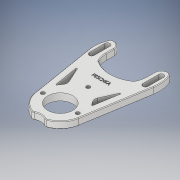
# Autodesk Inventor part: Motor Holder v3
Saved by Autodesk Inventor 2019.3 (Build 233278000, 278)
## iProperties
Created: 2019-03-01
Part Number: Motor Holder v3
Material: ABS Plastic
Document SubType Name: Modeling
Designer: Petar
Density: 1.06 g/cm^3
Appearance: Smooth - White
Mass: 26.5004 g
Surface Area: 70.5339 cm^2
Volume: 9.81495 cm^3
Author: Petar
Autodesk Inventor part; units mm, degrees
ref_plane "YZ Plane" through (0, 0, 0) normal (1, 0, 0) x (0, 1, 0)
ref_plane "XZ Plane" through (0, 0, 0) normal (0, 1, 0) x (-1, 0, 0)
ref_plane "XY Plane" through (0, 0, 0) normal (0, 0, 1) x (1, 0, 0)
sketch "Sketch1" plane through (0, 0, 0) normal (0, 1, 0) x (-1, 0, 0)
  line L0 (0, 0) -> (0, 52.2) construction
  circle A0 centre (0, 52.2) radius 10
  line L1 (16, -6.25) -> (16, 0)
  line L2 (21.2132, 18.9419) -> (21.2132, -15.0581) construction
  line L3 (-21.2132, 18) -> (-21.2132, -16) construction
  circle A1 centre (21.2132, 3.5) radius 1.75 construction
  circle A2 centre (21.2132, -3.5) radius 1.75 construction
  circle A3 centre (-21.2132, 3.5) radius 1.75 construction
  circle A4 centre (-21.2132, -3.5) radius 1.75 construction
  line L4 (-16, -6.25) -> (-16, 0)
  line L5 (21.2132, 6.25) -> (21.2132, -6.25) construction
  line L6 (19.2132, 6.25) -> (19.2132, -6.25)
  line L7 (23.2132, -6.25) -> (23.2132, 6.25)
  arc A5 (23.2132, 6.25) -> (19.2132, 6.25) centre (21.2132, 6.25) ccw
  arc A6 (19.2132, -6.25) -> (23.2132, -6.25) centre (21.2132, -6.25) ccw
  line L8 (-19.2132, 6.25) -> (-19.2132, -6.25)
  line L9 (-23.2132, -6.25) -> (-23.2132, 6.25)
  arc A7 (-19.2132, 6.25) -> (-23.2132, 6.25) centre (-21.2132, 6.25) ccw
  arc A8 (-23.2132, -6.25) -> (-19.2132, -6.25) centre (-21.2132, -6.25) ccw
  arc A9 (14.3275, 42.1515) -> (17.2664, 55.0496) centre (0, 52.2) ccw construction
  arc A10 (16, -6.25) -> (23.6156, -10.8766) centre (21.2132, -6.25) ccw
  arc A11 (-23.6156, -10.8766) -> (-16, -6.25) centre (-21.2132, -6.25) ccw
  line L10 (17.2664, 55.0496) -> (25.653, 4.2337)
  line L11 (-17.2664, 55.0496) -> (-25.653, 4.2337)
  circle A12 centre (0, 52.2) radius 13.75 construction
  circle A13 centre (9.7227, 61.9227) radius 1.5 construction
  circle A14 centre (9.7227, 42.4773) radius 1.5 construction
  line L12 (0, 52.2) -> (9.7227, 61.9227) construction
  line L13 (9.7227, 42.4773) -> (0, 52.2) construction
  circle A15 centre (-9.7227, 61.9227) radius 1.5 construction
  circle A16 centre (-9.7227, 42.4773) radius 1.5 construction
  circle A17 centre (13.75, 52.2) radius 1.5
  line L14 (13.75, 52.2) -> (0, 52.2) construction
  circle A18 centre (-13.75, 52.2) radius 1.5
  circle A19 centre (0, 30.2) radius 1.5
  line L15 (14.3275, 42.1515) -> (18.2235, 18.5446)
  arc A20 (17.2664, 55.0496) -> (-17.2664, 55.0496) centre (0, 52.2) ccw
  arc A21 (-17.2664, 55.0496) -> (-14.3275, 42.1515) centre (0, 52.2) ccw construction
  line L16 (-14.3275, 42.1515) -> (-18.2235, 18.5446)
  line L17 (5, 68.9705) -> (0, 65.95) construction
  line L18 (0, 65.95) -> (-5, 68.9705) construction
  spline S0 degree 2 poles (5, 68.9705) (0, 65.95) (-5, 68.9705) knots 1 1 1 2 2 2
  line L19 (5, 68.9705) -> (-5, 68.9705) construction
  line L20 (18.2235, 18.5446) -> (-18.2235, 18.5446) construction
  line L21 (18.2235, 18.5446) -> (11.2615, 33.9127)
  line L22 (14.3275, 42.1515) -> (11.6782, 38.374)
  arc A22 (11.6782, 38.374) -> (11.2615, 33.9127) centre (15.3793, 35.7782) ccw
  line L23 (-18.2235, 18.5446) -> (-11.2615, 33.9127)
  line L24 (-14.3275, 42.1515) -> (-11.6782, 38.374)
  arc A23 (-11.2615, 33.9127) -> (-11.6782, 38.374) centre (-15.3793, 35.7782) ccw
  line L25 (13.8322, 18.5446) -> (7.5291, 32.4581) construction
  line L26 (13.8322, 18.5446) -> (6.7139, 25.1182) construction
  line L27 (7.5291, 32.4581) -> (6.1396, 30.477) construction
  arc A24 (6.1396, 30.477) -> (6.7139, 25.1182) centre (9.4916, 28.126) ccw construction
  line L28 (-13.8322, 18.5446) -> (-7.5291, 32.4581) construction
  line L29 (-13.8322, 18.5446) -> (-6.7139, 25.1182) construction
  line L30 (-7.5291, 32.4581) -> (-6.1396, 30.477) construction
  arc A25 (-6.7139, 25.1182) -> (-6.1396, 30.477) centre (-9.4916, 28.126) ccw construction
  arc A26 (23.6156, -10.8766) -> (26, 0) centre (0, 0) ccw
  arc A27 (-23.6156, -10.8766) -> (23.6156, -10.8766) centre (0, 0) ccw construction
  arc A28 (-9.8788, 24.0502) -> (-25.653, 4.2337) centre (0, 0) ccw construction
  line L31 (21.2132, -11.4632) -> (-21.2132, -11.4632) construction
  line L32 (-21.2132, 69.7) -> (25, 69.7) construction
  line L33 (0, 65.95) -> (0, 62.2) construction
  arc A29 (13.761, 8.163) -> (-13.761, 8.163) centre (0, -11.5) ccw
  line L34 (13.761, 8.163) -> (-13.761, 8.163) construction
  arc A30 (16, 0) -> (13.761, 8.163) centre (0, 0) ccw
  arc A31 (-13.761, 8.163) -> (-16, 0) centre (0, 0) ccw
  arc A32 (26, 0) -> (25.653, 4.2337) centre (0, 0) ccw
  arc A33 (-26, 0) -> (-23.6156, -10.8766) centre (0, 0) ccw
  arc A34 (-25.653, 4.2337) -> (-26, 0) centre (0, 0) ccw
  arc A35 (25.653, 4.2337) -> (-11.7191, 23.2091) centre (0, 0) ccw construction
  line L35 (16, 0) -> (-16, 0) construction
  point P0 (21.2132, 0)
  point P1 (0, 12.5)
  dimension "d1" = 20
  dimension "d0" = 52.2
  dimension "d3" = 3.5
  dimension "d4" = 3.5
  dimension "d5" = 7
  dimension "d7" = 43
  dimension "d9" = 3.5
  dimension "d11" = 32
  dimension "d15" = 4
  dimension "d24" = 3
  dimension "d25" = 3
  dimension "d27" = 45
  dimension "d29" = 3
  dimension "d30" = 3
  dimension "d31" = 22
  dimension "d50" = 10
  dimension "d53" = 26
  dimension "d75" = 81.1632
  dimension "d76" = 7.5
  dimension "d77" = 3.75
  dimension "d81" = 6.25
  dimension "d82" = 12.5
  dimension "d85" = 5
  dimension "d86" = 4
  dimension "d98" = 15
  dimension "d99" = 24
  constraints: 70 end point, 59 point on circle, 35 centre point, 26 symmetric about line, 19 tangent, 13 point on line, 7 coincident, 5 horizontal, 5 vertical, 3 parallel, 2 perpendicular, 1 collinear, 1 midpoint, 1 vertical alignment, 16 other
  measures "d0" distance of L0.start L0.end
  measures "d3" diameter of A1
  measures "d4" diameter of A2
  measures "d5" distance of A2.centre A1.centre
  measures "d7" distance of A2.centre A3.centre
  measures "d9" vertical distance of L0.start A1.centre
  measures "d11" distance between parallel lines of L4 L1
  measures "d15" distance between parallel lines of L6 L7
  measures "d24" diameter of A13
  measures "d25" diameter of A14
  measures "d27" angle of L0 L13
  measures "d29" diameter of A17
  measures "d30" diameter of A19
  measures "d31" distance of L0.end A19.centre
  measures "d50" distance of L17.start L18.end
  measures "d53" radius of A26
  measures "d75" distance between parallel lines of L31 L32
  measures "d81" vertical distance of L5.start point (0, 12.5)
  measures "d82" distance of L5.end L5.start
  measures "d85" distance between parallel lines of L10 L15
  measures "d86" distance between parallel lines of L21 L25
  measures "d98" angle of L15 L21
  measures "d99" radius of A29
extrude "Extrusion3" add sketch "Sketch1" along normal blind 5.5 contours L1 A30 A29 A31 L4 A11 A33 A34 L11 A20 S0 L10 A32 A26 A10
thread "Thread1" size "M3x0.5" class "6H" standard "ANSI Metric M Profile" full length
thread "Thread2" size "M3x0.5" class "6H" standard "ANSI Metric M Profile" full length
thread "Thread3" size "M3x0.5" class "6H" standard "ANSI Metric M Profile" full length
sketch "Sketch3" plane through (0, 5.5, 0) normal (0, 1, 0) x (1, 0, 0)
  line L0 (-7.5, -17.2) -> (7.5, -17.2) construction
  line L1 (7.5, -17.2) -> (7.5, -22.2) construction
  line L2 (7.5, -22.2) -> (-7.5, -22.2) construction
  line L3 (-7.5, -22.2) -> (-7.5, -17.2) construction
  line L4 (0, 0) -> (0, -60) construction
  circle A0 centre (0, -30.2) radius 1.5 projected
  spline S0 degree 2 poles (-5.044, -19.1957) (-5.044, -19.3604) (-5.1613, -19.6568) (-5.2663, -19.7597) knots 0 0 0 1 2 2 2
  spline S1 degree 2 poles (-5.2663, -19.7597) (-5.398, -19.8894) (-5.7541, -20.0232) (-6.0258, -20.0232) knots 0 0 0 1 2 2 2
  line L5 (-6.0258, -20.0232) -> (-6.3119, -20.0232)
  line L6 (-6.3119, -20.0232) -> (-6.3119, -20.97)
  line L7 (-6.3119, -20.97) -> (-6.6495, -20.97)
  line L8 (-6.6495, -20.97) -> (-6.6495, -18.43)
  line L9 (-6.6495, -18.43) -> (-6.0114, -18.43)
  spline S2 degree 2 poles (-6.0114, -18.43) (-5.785, -18.43) (-5.468, -18.5041) (-5.3466, -18.5885) knots 0 0 0 1 2 2 2
  spline S3 degree 2 poles (-5.3466, -18.5885) (-5.2045, -18.6852) (-5.044, -18.9837) (-5.044, -19.1957) knots 0 0 0 1 2 2 2
  spline S4 degree 2 poles (-5.396, -19.206) (-5.396, -19.0743) (-5.4865, -18.8808) (-5.5791, -18.819) knots 0 0 0 1 2 2 2
  spline S5 degree 2 poles (-5.5791, -18.819) (-5.6594, -18.7655) (-5.8735, -18.7223) (-6.032, -18.7223) knots 0 0 0 1 2 2 2
  line L10 (-6.032, -18.7223) -> (-6.3119, -18.7223)
  line L11 (-6.3119, -18.7223) -> (-6.3119, -19.735)
  line L12 (-6.3119, -19.735) -> (-6.0814, -19.735)
  spline S6 degree 2 poles (-6.0814, -19.735) (-5.8756, -19.735) (-5.6224, -19.6691) (-5.54, -19.5827) knots 0 0 0 1 2 2 2
  spline S7 degree 2 poles (-5.54, -19.5827) (-5.4639, -19.5065) (-5.396, -19.3274) (-5.396, -19.206) knots 0 0 0 1 2 2 2
  line L13 (-3.8378, -20.97) -> (-4.8217, -20.97)
  line L14 (-4.8217, -20.97) -> (-4.8217, -20.7106)
  line L15 (-4.8217, -20.7106) -> (-4.4985, -20.7106)
  line L16 (-4.4985, -20.7106) -> (-4.4985, -18.6894)
  line L17 (-4.4985, -18.6894) -> (-4.8217, -18.6894)
  line L18 (-4.8217, -18.6894) -> (-4.8217, -18.43)
  line L19 (-4.8217, -18.43) -> (-3.8378, -18.43)
  line L20 (-3.8378, -18.43) -> (-3.8378, -18.6894)
  line L21 (-3.8378, -18.6894) -> (-4.1609, -18.6894)
  line L22 (-4.1609, -18.6894) -> (-4.1609, -20.7106)
  line L23 (-4.1609, -20.7106) -> (-3.8378, -20.7106)
  line L24 (-3.8378, -20.7106) -> (-3.8378, -20.97)
  spline S8 degree 2 poles (-2.7119, -21.0153) (-2.9877, -21.0153) (-3.3747, -20.9) (-3.5455, -20.8177) knots 0 0 0 1 2 2 2
  line L25 (-3.5455, -20.8177) -> (-3.5455, -20.3937)
  line L26 (-3.5455, -20.3937) -> (-3.5208, -20.3937)
  spline S9 degree 2 poles (-3.5208, -20.3937) (-3.3541, -20.5501) (-2.9321, -20.723) (-2.7366, -20.723) knots 0 0 0 1 2 2 2
  spline S10 degree 2 poles (-2.7366, -20.723) (-2.4566, -20.723) (-2.1705, -20.4904) (-2.1705, -20.299) knots 0 0 0 1 2 2 2
  spline S11 degree 2 poles (-2.1705, -20.299) (-2.1705, -20.1467) (-2.3208, -19.9573) (-2.4834, -19.91) knots 0 0 0 1 2 2 2
  spline S12 degree 2 poles (-2.4834, -19.91) (-2.6007, -19.877) (-2.7963, -19.8317) (-2.9424, -19.7947) knots 0 0 0 1 2 2 2
  spline S13 degree 2 poles (-2.9424, -19.7947) (-3.0741, -19.7597) (-3.282, -19.6547) (-3.3623, -19.5703) knots 0 0 0 1 2 2 2
  spline S14 degree 2 poles (-3.3623, -19.5703) (-3.4405, -19.4859) (-3.527, -19.2595) (-3.527, -19.1113) knots 0 0 0 1 2 2 2
  spline S15 degree 2 poles (-3.527, -19.1113) (-3.527, -18.8026) (-3.0453, -18.3847) (-2.6728, -18.3847) knots 0 0 0 1 2 2 2
  spline S16 degree 2 poles (-2.6728, -18.3847) (-2.4587, -18.3847) (-2.08, -18.4691) (-1.9174, -18.5494) knots 0 0 0 1 2 2 2
  line L27 (-1.9174, -18.5494) -> (-1.9174, -18.9528)
  line L28 (-1.9174, -18.9528) -> (-1.9421, -18.9528)
  spline S17 degree 2 poles (-1.9421, -18.9528) (-2.0635, -18.8417) (-2.4422, -18.677) (-2.6501, -18.677) knots 0 0 0 1 2 2 2
  spline S18 degree 2 poles (-2.6501, -18.677) (-2.8848, -18.677) (-3.175, -18.8972) (-3.175, -19.0763) knots 0 0 0 1 2 2 2
  spline S19 degree 2 poles (-3.175, -19.0763) (-3.175, -19.2369) (-3.0042, -19.4283) (-2.8436, -19.4715) knots 0 0 0 1 2 2 2
  spline S20 degree 2 poles (-2.8436, -19.4715) (-2.7366, -19.5003) (-2.4258, -19.5744) (-2.3228, -19.6053) knots 0 0 0 1 2 2 2
  spline S21 degree 2 poles (-2.3228, -19.6053) (-2.0614, -19.6856) (-1.8185, -20.0088) (-1.8185, -20.2455) knots 0 0 0 1 2 2 2
  spline S22 degree 2 poles (-1.8185, -20.2455) (-1.8185, -20.3957) (-1.94, -20.6839) (-2.0491, -20.7847) knots 0 0 0 1 2 2 2
  spline S23 degree 2 poles (-2.0491, -20.7847) (-2.1705, -20.8959) (-2.4793, -21.0153) (-2.7119, -21.0153) knots 0 0 0 1 2 2 2
  spline S24 degree 2 poles (-0.4827, -21.0153) (-0.7297, -21.0153) (-1.1475, -20.8486) (-1.2998, -20.6818) knots 0 0 0 1 2 2 2
  spline S25 degree 2 poles (-1.2998, -20.6818) (-1.4522, -20.5172) (-1.6189, -20.0232) (-1.6189, -19.7021) knots 0 0 0 1 2 2 2
  spline S26 degree 2 poles (-1.6189, -19.7021) (-1.6189, -19.383) (-1.4563, -18.9096) (-1.3019, -18.7346) knots 0 0 0 1 2 2 2
  spline S27 degree 2 poles (-1.3019, -18.7346) (-1.1496, -18.5638) (-0.7338, -18.3847) (-0.4765, -18.3847) knots 0 0 0 1 2 2 2
  spline S28 degree 2 poles (-0.4765, -18.3847) (-0.3489, -18.3847) (-0.1245, -18.4218) (-0.0298, -18.4506) knots 0 0 0 1 2 2 2
  spline S29 degree 2 poles (-0.0298, -18.4506) (0.0525, -18.4773) (0.2233, -18.5535) (0.3077, -18.5988) knots 0 0 0 1 2 2 2
  line L29 (0.3077, -18.5988) -> (0.3077, -19.0063)
  line L30 (0.3077, -19.0063) -> (0.281, -19.0063)
  spline S30 degree 2 poles (0.281, -19.0063) (0.2357, -18.9652) (0.0957, -18.8499) (-0.0051, -18.7943) knots 0 0 0 1 2 2 2
  spline S31 degree 2 poles (-0.0051, -18.7943) (-0.1019, -18.7408) (-0.3304, -18.6729) (-0.4786, -18.6729) knots 0 0 0 1 2 2 2
  spline S32 degree 2 poles (-0.4786, -18.6729) (-0.6412, -18.6729) (-0.9314, -18.8067) (-1.0405, -18.9343) knots 0 0 0 1 2 2 2
  spline S33 degree 2 poles (-1.0405, -18.9343) (-1.1475, -19.064) (-1.2669, -19.4571) (-1.2669, -19.7021) knots 0 0 0 1 2 2 2
  spline S34 degree 2 poles (-1.2669, -19.7021) (-1.2669, -19.9635) (-1.1414, -20.3401) (-1.0323, -20.4698) knots 0 0 0 1 2 2 2
  spline S35 degree 2 poles (-1.0323, -20.4698) (-0.9252, -20.5954) (-0.6391, -20.723) (-0.4786, -20.723) knots 0 0 0 1 2 2 2
  spline S36 degree 2 poles (-0.4786, -20.723) (-0.3324, -20.723) (-0.0834, -20.651) (0.0134, -20.5974) knots 0 0 0 1 2 2 2
  spline S37 degree 2 poles (0.0134, -20.5974) (0.106, -20.5439) (0.2439, -20.4328) (0.283, -20.3937) knots 0 0 0 1 2 2 2
  line L31 (0.283, -20.3937) -> (0.3077, -20.3937)
  line L32 (0.3077, -20.3937) -> (0.3077, -20.7971)
  spline S38 degree 2 poles (0.3077, -20.7971) (0.2233, -20.8362) (0.0751, -20.9082) (-0.0298, -20.9412) knots 0 0 0 1 2 2 2
  spline S39 degree 2 poles (-0.0298, -20.9412) (-0.141, -20.9782) (-0.3304, -21.0153) (-0.4827, -21.0153) knots 0 0 0 1 2 2 2
  line L33 (2.4669, -20.97) -> (2.1294, -20.97)
  line L34 (2.1294, -20.97) -> (2.1294, -19.7268)
  line L35 (2.1294, -19.7268) -> (0.9602, -19.7268)
  line L36 (0.9602, -19.7268) -> (0.9602, -20.97)
  line L37 (0.9602, -20.97) -> (0.6226, -20.97)
  line L38 (0.6226, -20.97) -> (0.6226, -18.43)
  line L39 (0.6226, -18.43) -> (0.9602, -18.43)
  line L40 (0.9602, -18.43) -> (0.9602, -19.4262)
  line L41 (0.9602, -19.4262) -> (2.1294, -19.4262)
  line L42 (2.1294, -19.4262) -> (2.1294, -18.43)
  line L43 (2.1294, -18.43) -> (2.4669, -18.43)
  line L44 (2.4669, -18.43) -> (2.4669, -20.97)
  line L45 (4.834, -20.97) -> (4.3956, -20.97)
  line L46 (4.3956, -20.97) -> (3.4673, -19.7885)
  line L47 (3.4673, -19.7885) -> (3.3191, -19.9552)
  line L48 (3.3191, -19.9552) -> (3.3191, -20.97)
  line L49 (3.3191, -20.97) -> (2.9815, -20.97)
  line L50 (2.9815, -20.97) -> (2.9815, -18.43)
  line L51 (2.9815, -18.43) -> (3.3191, -18.43)
  line L52 (3.3191, -18.43) -> (3.3191, -19.5971)
  line L53 (3.3191, -19.5971) -> (4.3606, -18.43)
  line L54 (4.3606, -18.43) -> (4.7723, -18.43)
  line L55 (4.7723, -18.43) -> (3.7205, -19.5641)
  line L56 (3.7205, -19.5641) -> (4.834, -20.97)
  line L57 (4.762, -20.97) -> (5.6183, -18.43)
  line L58 (5.6183, -18.43) -> (6.034, -18.43)
  line L59 (6.034, -18.43) -> (6.8903, -20.97)
  line L60 (6.8903, -20.97) -> (6.5342, -20.97)
  line L61 (6.5342, -20.97) -> (6.3037, -20.2599)
  line L62 (6.3037, -20.2599) -> (5.3342, -20.2599)
  line L63 (5.3342, -20.2599) -> (5.1037, -20.97)
  line L64 (5.1037, -20.97) -> (4.762, -20.97)
  line L65 (6.2111, -19.9717) -> (5.8179, -18.7758)
  line L66 (5.8179, -18.7758) -> (5.4268, -19.9717)
  line L67 (5.4268, -19.9717) -> (6.2111, -19.9717)
  dimension "d68" = 8
  dimension "d69" = 5
  dimension "d70" = 15
  constraints: 2 end point, 1 vertical, 3 other
  measures "d68" distance from line of L2 A0.centre
  measures "d69" distance between parallel lines of L0 L2
  measures "d70" distance between parallel lines of L3 L1
emboss "Emboss1" sketch "Sketch3" operation cut depth 0.2 direction (0, -1, 0) contours S0 S1 L5 L6 L7 L8 L9 S2 S3 | L13 L14 L15 L16 L17 L18 L19 L20 L21 L22 L23 L24 | S8 L25 L26 S9 S10 S11 S12 S13 S14 S15 S16 L27 L28 S17 S18 S19 S20 S21 S22 S23 | S24 S25 S26 S27 S28 S29 L29 L30 S30 S31 S32 S33 S34 S35 S36 S37 L31 L32 S38 S39 | L33 L34 L35 L36 L37 L38 L39 L40 L41 L42 L43 L44 | L45 L57 L56 | L56 L57 L58 L59 L60 L61 L62 L63 L64 | L45 L46 L47 L48 L49 L50 L51 L52 L53 L54 L55 L56 L57
sketch "Sketch4" plane through (0, 0, 0) normal (0, -1, 0) x (1, 0, 0)
  circle A0 centre (0, 30.2) radius 1.5 projected
  line L0 (7.5, 17.2) -> (-7.5, 17.2) construction
  line L1 (-7.5, 17.2) -> (-7.5, 22.2) construction
  line L2 (-7.5, 22.2) -> (7.5, 22.2) construction
  line L3 (7.5, 22.2) -> (7.5, 17.2) construction
  spline S0 degree 2 poles (5.044, 19.1957) (5.044, 19.3604) (5.1613, 19.6568) (5.2663, 19.7597) knots 0 0 0 1 2 2 2
  spline S1 degree 2 poles (5.2663, 19.7597) (5.398, 19.8894) (5.7541, 20.0232) (6.0258, 20.0232) knots 0 0 0 1 2 2 2
  line L4 (6.0258, 20.0232) -> (6.3119, 20.0232)
  line L5 (6.3119, 20.0232) -> (6.3119, 20.97)
  line L6 (6.3119, 20.97) -> (6.6495, 20.97)
  line L7 (6.6495, 20.97) -> (6.6495, 18.43)
  line L8 (6.6495, 18.43) -> (6.0114, 18.43)
  spline S2 degree 2 poles (6.0114, 18.43) (5.785, 18.43) (5.468, 18.5041) (5.3466, 18.5885) knots 0 0 0 1 2 2 2
  spline S3 degree 2 poles (5.3466, 18.5885) (5.2045, 18.6852) (5.044, 18.9837) (5.044, 19.1957) knots 0 0 0 1 2 2 2
  spline S4 degree 2 poles (5.396, 19.206) (5.396, 19.0743) (5.4865, 18.8808) (5.5791, 18.819) knots 0 0 0 1 2 2 2
  spline S5 degree 2 poles (5.5791, 18.819) (5.6594, 18.7655) (5.8735, 18.7223) (6.032, 18.7223) knots 0 0 0 1 2 2 2
  line L9 (6.032, 18.7223) -> (6.3119, 18.7223)
  line L10 (6.3119, 18.7223) -> (6.3119, 19.735)
  line L11 (6.3119, 19.735) -> (6.0814, 19.735)
  spline S6 degree 2 poles (6.0814, 19.735) (5.8756, 19.735) (5.6224, 19.6691) (5.54, 19.5827) knots 0 0 0 1 2 2 2
  spline S7 degree 2 poles (5.54, 19.5827) (5.4639, 19.5065) (5.396, 19.3274) (5.396, 19.206) knots 0 0 0 1 2 2 2
  line L12 (3.8378, 20.97) -> (4.8217, 20.97)
  line L13 (4.8217, 20.97) -> (4.8217, 20.7106)
  line L14 (4.8217, 20.7106) -> (4.4985, 20.7106)
  line L15 (4.4985, 20.7106) -> (4.4985, 18.6894)
  line L16 (4.4985, 18.6894) -> (4.8217, 18.6894)
  line L17 (4.8217, 18.6894) -> (4.8217, 18.43)
  line L18 (4.8217, 18.43) -> (3.8378, 18.43)
  line L19 (3.8378, 18.43) -> (3.8378, 18.6894)
  line L20 (3.8378, 18.6894) -> (4.1609, 18.6894)
  line L21 (4.1609, 18.6894) -> (4.1609, 20.7106)
  line L22 (4.1609, 20.7106) -> (3.8378, 20.7106)
  line L23 (3.8378, 20.7106) -> (3.8378, 20.97)
  spline S8 degree 2 poles (2.7119, 21.0153) (2.9877, 21.0153) (3.3747, 20.9) (3.5455, 20.8177) knots 0 0 0 1 2 2 2
  line L24 (3.5455, 20.8177) -> (3.5455, 20.3937)
  line L25 (3.5455, 20.3937) -> (3.5208, 20.3937)
  spline S9 degree 2 poles (3.5208, 20.3937) (3.3541, 20.5501) (2.9321, 20.723) (2.7366, 20.723) knots 0 0 0 1 2 2 2
  spline S10 degree 2 poles (2.7366, 20.723) (2.4566, 20.723) (2.1705, 20.4904) (2.1705, 20.299) knots 0 0 0 1 2 2 2
  spline S11 degree 2 poles (2.1705, 20.299) (2.1705, 20.1467) (2.3208, 19.9573) (2.4834, 19.91) knots 0 0 0 1 2 2 2
  spline S12 degree 2 poles (2.4834, 19.91) (2.6007, 19.877) (2.7963, 19.8317) (2.9424, 19.7947) knots 0 0 0 1 2 2 2
  spline S13 degree 2 poles (2.9424, 19.7947) (3.0741, 19.7597) (3.282, 19.6547) (3.3623, 19.5703) knots 0 0 0 1 2 2 2
  spline S14 degree 2 poles (3.3623, 19.5703) (3.4405, 19.4859) (3.527, 19.2595) (3.527, 19.1113) knots 0 0 0 1 2 2 2
  spline S15 degree 2 poles (3.527, 19.1113) (3.527, 18.8026) (3.0453, 18.3847) (2.6728, 18.3847) knots 0 0 0 1 2 2 2
  spline S16 degree 2 poles (2.6728, 18.3847) (2.4587, 18.3847) (2.08, 18.4691) (1.9174, 18.5494) knots 0 0 0 1 2 2 2
  line L26 (1.9174, 18.5494) -> (1.9174, 18.9528)
  line L27 (1.9174, 18.9528) -> (1.9421, 18.9528)
  spline S17 degree 2 poles (1.9421, 18.9528) (2.0635, 18.8417) (2.4422, 18.677) (2.6501, 18.677) knots 0 0 0 1 2 2 2
  spline S18 degree 2 poles (2.6501, 18.677) (2.8848, 18.677) (3.175, 18.8972) (3.175, 19.0763) knots 0 0 0 1 2 2 2
  spline S19 degree 2 poles (3.175, 19.0763) (3.175, 19.2369) (3.0042, 19.4283) (2.8436, 19.4715) knots 0 0 0 1 2 2 2
  spline S20 degree 2 poles (2.8436, 19.4715) (2.7366, 19.5003) (2.4258, 19.5744) (2.3228, 19.6053) knots 0 0 0 1 2 2 2
  spline S21 degree 2 poles (2.3228, 19.6053) (2.0614, 19.6856) (1.8185, 20.0088) (1.8185, 20.2455) knots 0 0 0 1 2 2 2
  spline S22 degree 2 poles (1.8185, 20.2455) (1.8185, 20.3957) (1.94, 20.6839) (2.0491, 20.7847) knots 0 0 0 1 2 2 2
  spline S23 degree 2 poles (2.0491, 20.7847) (2.1705, 20.8959) (2.4793, 21.0153) (2.7119, 21.0153) knots 0 0 0 1 2 2 2
  spline S24 degree 2 poles (0.4827, 21.0153) (0.7297, 21.0153) (1.1475, 20.8486) (1.2998, 20.6818) knots 0 0 0 1 2 2 2
  spline S25 degree 2 poles (1.2998, 20.6818) (1.4522, 20.5172) (1.6189, 20.0232) (1.6189, 19.7021) knots 0 0 0 1 2 2 2
  spline S26 degree 2 poles (1.6189, 19.7021) (1.6189, 19.383) (1.4563, 18.9096) (1.3019, 18.7346) knots 0 0 0 1 2 2 2
  spline S27 degree 2 poles (1.3019, 18.7346) (1.1496, 18.5638) (0.7338, 18.3847) (0.4765, 18.3847) knots 0 0 0 1 2 2 2
  spline S28 degree 2 poles (0.4765, 18.3847) (0.3489, 18.3847) (0.1245, 18.4218) (0.0298, 18.4506) knots 0 0 0 1 2 2 2
  spline S29 degree 2 poles (0.0298, 18.4506) (-0.0525, 18.4773) (-0.2233, 18.5535) (-0.3077, 18.5988) knots 0 0 0 1 2 2 2
  line L28 (-0.3077, 18.5988) -> (-0.3077, 19.0063)
  line L29 (-0.3077, 19.0063) -> (-0.281, 19.0063)
  spline S30 degree 2 poles (-0.281, 19.0063) (-0.2357, 18.9652) (-0.0957, 18.8499) (0.0051, 18.7943) knots 0 0 0 1 2 2 2
  spline S31 degree 2 poles (0.0051, 18.7943) (0.1019, 18.7408) (0.3304, 18.6729) (0.4786, 18.6729) knots 0 0 0 1 2 2 2
  spline S32 degree 2 poles (0.4786, 18.6729) (0.6412, 18.6729) (0.9314, 18.8067) (1.0405, 18.9343) knots 0 0 0 1 2 2 2
  spline S33 degree 2 poles (1.0405, 18.9343) (1.1475, 19.064) (1.2669, 19.4571) (1.2669, 19.7021) knots 0 0 0 1 2 2 2
  spline S34 degree 2 poles (1.2669, 19.7021) (1.2669, 19.9635) (1.1414, 20.3401) (1.0323, 20.4698) knots 0 0 0 1 2 2 2
  spline S35 degree 2 poles (1.0323, 20.4698) (0.9252, 20.5954) (0.6391, 20.723) (0.4786, 20.723) knots 0 0 0 1 2 2 2
  spline S36 degree 2 poles (0.4786, 20.723) (0.3324, 20.723) (0.0834, 20.651) (-0.0134, 20.5974) knots 0 0 0 1 2 2 2
  spline S37 degree 2 poles (-0.0134, 20.5974) (-0.106, 20.5439) (-0.2439, 20.4328) (-0.283, 20.3937) knots 0 0 0 1 2 2 2
  line L30 (-0.283, 20.3937) -> (-0.3077, 20.3937)
  line L31 (-0.3077, 20.3937) -> (-0.3077, 20.7971)
  spline S38 degree 2 poles (-0.3077, 20.7971) (-0.2233, 20.8362) (-0.0751, 20.9082) (0.0298, 20.9412) knots 0 0 0 1 2 2 2
  spline S39 degree 2 poles (0.0298, 20.9412) (0.141, 20.9782) (0.3304, 21.0153) (0.4827, 21.0153) knots 0 0 0 1 2 2 2
  line L32 (-2.4669, 20.97) -> (-2.1294, 20.97)
  line L33 (-2.1294, 20.97) -> (-2.1294, 19.7268)
  line L34 (-2.1294, 19.7268) -> (-0.9602, 19.7268)
  line L35 (-0.9602, 19.7268) -> (-0.9602, 20.97)
  line L36 (-0.9602, 20.97) -> (-0.6226, 20.97)
  line L37 (-0.6226, 20.97) -> (-0.6226, 18.43)
  line L38 (-0.6226, 18.43) -> (-0.9602, 18.43)
  line L39 (-0.9602, 18.43) -> (-0.9602, 19.4262)
  line L40 (-0.9602, 19.4262) -> (-2.1294, 19.4262)
  line L41 (-2.1294, 19.4262) -> (-2.1294, 18.43)
  line L42 (-2.1294, 18.43) -> (-2.4669, 18.43)
  line L43 (-2.4669, 18.43) -> (-2.4669, 20.97)
  line L44 (-4.834, 20.97) -> (-4.3956, 20.97)
  line L45 (-4.3956, 20.97) -> (-3.4673, 19.7885)
  line L46 (-3.4673, 19.7885) -> (-3.3191, 19.9552)
  line L47 (-3.3191, 19.9552) -> (-3.3191, 20.97)
  line L48 (-3.3191, 20.97) -> (-2.9815, 20.97)
  line L49 (-2.9815, 20.97) -> (-2.9815, 18.43)
  line L50 (-2.9815, 18.43) -> (-3.3191, 18.43)
  line L51 (-3.3191, 18.43) -> (-3.3191, 19.5971)
  line L52 (-3.3191, 19.5971) -> (-4.3606, 18.43)
  line L53 (-4.3606, 18.43) -> (-4.7723, 18.43)
  line L54 (-4.7723, 18.43) -> (-3.7205, 19.5641)
  line L55 (-3.7205, 19.5641) -> (-4.834, 20.97)
  line L56 (-4.762, 20.97) -> (-5.6183, 18.43)
  line L57 (-5.6183, 18.43) -> (-6.034, 18.43)
  line L58 (-6.034, 18.43) -> (-6.8903, 20.97)
  line L59 (-6.8903, 20.97) -> (-6.5342, 20.97)
  line L60 (-6.5342, 20.97) -> (-6.3037, 20.2599)
  line L61 (-6.3037, 20.2599) -> (-5.3342, 20.2599)
  line L62 (-5.3342, 20.2599) -> (-5.1037, 20.97)
  line L63 (-5.1037, 20.97) -> (-4.762, 20.97)
  line L64 (-6.2111, 19.9717) -> (-5.8179, 18.7758)
  line L65 (-5.8179, 18.7758) -> (-5.4268, 19.9717)
  line L66 (-5.4268, 19.9717) -> (-6.2111, 19.9717)
  dimension "d67" = 8
  dimension "d71" = 5
  dimension "d72" = 15
  constraints: 2 other
  measures "d67" distance from line of L2 A0.centre
  measures "d71" distance between parallel lines of L2 L0
  measures "d72" distance between parallel lines of L3 L1
emboss "Emboss2" sketch "Sketch4" operation cut depth 0.2 direction (0, 1, 0) contours S0 S1 L4 L5 L6 L7 L8 S2 S3 | L12 L13 L14 L15 L16 L17 L18 L19 L20 L21 L22 L23 | S8 L24 L25 S9 S10 S11 S12 S13 S14 S15 S16 L26 L27 S17 S18 S19 S20 S21 S22 S23 | S24 S25 S26 S27 S28 S29 L28 L29 S30 S31 S32 S33 S34 S35 S36 S37 L30 L31 S38 S39 | L32 L33 L34 L35 L36 L37 L38 L39 L40 L41 L42 L43 | L44 L56 L55 | L55 L56 L57 L58 L59 L60 L61 L62 L63 | L44 L45 L46 L47 L48 L49 L50 L51 L52 L53 L54 L55 L56
fillet "Fillet3" radius 0.5 4 edges at (-18.2235, 2.75, 18.5446) (-14.3275, 2.75, 42.1515) (14.3275, 2.75, 42.1515) (18.2235, 2.75, 18.5446)
fillet "Fillet5" radius 2 6 edges at (-5, 2.75, 68.9705) (5, 2.75, 68.9705) (23.6156, 2.75, -10.8766) (-23.6156, 2.75, -10.8766) (-13.761, 2.75, 8.163) (13.761, 2.75, 8.163)
chamfer "Chamfer3" distance 0.5 angle 45 40 edges at (13.4331, 5.5, 63.4162) (21.4597, 5.5, 29.6417) (25.8193, 5.5, -3.0604) (23.4392, 5.5, -10.8298) (18.0833, 5.5, -10.419) (16, 5.5, -3.125) (15.4929, 5.5, 3.9962) (13.7269, 5.5, 8.124) (0, 5.5, 12.5) (5.0769, 5.5, 68.7928) (0, 5.5, 67.4603) (-5.0769, 5.5, 68.7928) (-13.4331, 5.5, 63.4162) (-21.4597, 5.5, 29.6417) (-25.8193, 5.5, -3.0604) (-23.4392, 5.5, -10.8298) (-18.0833, 5.5, -10.419) (-16, 5.5, -3.125) (-15.4929, 5.5, 3.9962) (-13.7269, 5.5, 8.124) (0, 0, 67.4603) (5.0769, 0, 68.7928) (13.4331, 0, 63.4162) (21.4597, 0, 29.6417) (25.8193, 0, -3.0604) (23.4392, 0, -10.8298) (18.0833, 0, -10.419) (16, 0, -3.125) (15.4929, 0, 3.9962) (13.7269, 0, 8.124) (0, 0, 12.5) (-5.0769, 0, 68.7928) (-13.4331, 0, 63.4162) (-21.4597, 0, 29.6417) (-25.8193, 0, -3.0604) (-23.4392, 0, -10.8298) (-18.0833, 0, -10.419) (-16, 0, -3.125) (-15.4929, 0, 3.9962) (-13.7269, 0, 8.124)
sketch "Center Lines" plane through (0, 5.5, 0) normal (0, 1, 0) x (1, 0, 0)
  arc A0 (-23.2132, -6.25) -> (-19.2132, -6.25) centre (-21.2132, -6.25) ccw construction
  line L0 (-23.2132, -6.25) -> (-23.2132, 6.25) construction
  arc A1 (-19.2132, 6.25) -> (-23.2132, 6.25) centre (-21.2132, 6.25) ccw construction
  line L1 (-19.2132, 6.25) -> (-19.2132, -6.25) construction
  line L2 (-21.2132, -6.25) -> (-21.2132, 6.25) construction
  line L3 (19.2132, -6.25) -> (19.2132, 6.25) construction
  arc A2 (19.2132, -6.25) -> (23.2132, -6.25) centre (21.2132, -6.25) ccw construction
  line L4 (23.2132, 6.25) -> (23.2132, -6.25) construction
  arc A3 (23.2132, 6.25) -> (19.2132, 6.25) centre (21.2132, 6.25) ccw construction
  line L5 (21.2132, -6.25) -> (21.2132, 6.25) construction
  constraints: 4 end point, 2 vertical
body "Solid3"
